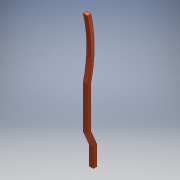
# Autodesk Inventor part: pins2
Saved by Autodesk Inventor 2016 (Build 200138000, 138)
## iProperties
Created: 2016-07-08
Part Number: pins2
Material: Copper
Document SubType Name: Modeling
Designer: Jonathan
Density: 8.94 g/cm^3
Appearance: Copper - Satin
Author: Jonathan
Autodesk Inventor part; units mm, degrees
ref_plane "YZ Plane" through (0, 0, 0) normal (1, 0, 0) x (0, 1, 0)
ref_plane "XZ Plane" through (0, 0, 0) normal (0, 1, 0) x (-1, 0, 0)
ref_plane "XY Plane" through (0, 0, 0) normal (0, 0, 1) x (1, 0, 0)
sketch "Sketch1" plane through (0, 0, 0) normal (1, 0, 0) x (0, 1, 0)
  line L0 (7.85, -6.14) -> (7.85, -5.0064)
  line L1 (7.85, -5.0064) -> (7.5, -4.1799)
  line L2 (7.5, -4.1799) -> (7.5, -1.7436)
  arc A0 (7.5, -1.7436) -> (7.5, 1.7436) centre (0, 0) ccw
  line L3 (7.5, 1.7436) -> (7.2945, 1.7436)
  arc A1 (7.3, -1.7205) -> (7.2945, 1.7436) centre (0, 0) ccw
  line L4 (7.3, -1.7205) -> (7.3, -4.2205)
  line L5 (7.3, -4.2205) -> (7.65, -5.047)
  line L6 (7.65, -5.047) -> (7.65, -6.14)
  line L7 (7.65, -6.14) -> (7.85, -6.14)
  line L8 (7.7, 1) -> (7.7, -1) construction
  point P0 (7.3973, 1.7436)
  point P1 (7.7, 0)
  point P2 (7.75, -6.14)
  dimension "d19" = 0.2
  dimension "d20" = 0.2
  dimension "d21" = 0.2
  dimension "d25" = 6.75
  dimension "d26" = 1.093
  dimension "d27" = 2.5
  dimension "d29" = 2
  dimension "d31" = 7.5
  dimension "d35" = 0.2
  dimension "d38" = 0.4
  dimension "d39" = 0.25
  constraints: 18 end point, 5 point on circle, 3 midpoint, 3 vertical, 2 centre point, 2 parallel, 1 coincident, 1 concentric, 1 horizontal, 1 perpendicular, 1 tangent
  measures "d19" distance between parallel lines of L6 L0
  measures "d20" distance between parallel lines of L5 L1
  measures "d21" distance between parallel lines of L4 L2
  measures "d25" distance from line of L0.end L3
  measures "d26" distance from line of L7 L5.end
  measures "d27" distance of L4.start L4.end
  measures "d29" distance of L8.start L8.end
  measures "d31" radius of A1
  measures "d35" radial gap between concentric circles of A1 A0
  measures "d38" distance between parallel lines of L4 L8
  measures "d39" distance from line of point (7.75, -6.14) L2
extrude "Extrusion1" add sketch "Sketch1" along normal mid plane 0.25
body "Solid1"
